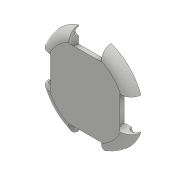
# Autodesk Inventor part: wheel_cover_in
Saved by Autodesk Inventor 2017 (Build 210142000, 142)
## iProperties
Created: 2018-10-27
Part Number: wheel_cover_in
Material: Generic
Document SubType Name: Modeling
Designer: mfans
Density: 1 g/cm^3
Appearance: Default
Author: mfans
Autodesk Inventor part; units mm, degrees
ref_plane "YZ Plane" through (0, 0, 0) normal (1, 0, 0) x (0, 1, 0)
ref_plane "XZ Plane" through (0, 0, 0) normal (0, 1, 0) x (-1, 0, 0)
ref_plane "XY Plane" through (0, 0, 0) normal (0, 0, 1) x (1, 0, 0)
sketch "Sketch1" plane through (0, 0, 0) normal (0, 1, 0) x (-1, 0, 0)
  circle A0 centre (0, 0) radius 30
  dimension "d0" = 60
  constraints: 1 centre point, 1 coincident
  measures "d0" diameter of A0
extrude "Extrusion1" add sketch "Sketch1" against normal blind 6
sketch "Sketch2" plane through (0, 0, 0) normal (0, 1, 0) x (1, 0, 0)
  line L0 (-10, -18) -> (10, -18)
  line L1 (10, -32) -> (-10, -32)
  line L2 (-10, -18) -> (10, -32) construction
  line L3 (10, -18) -> (-10, -32) construction
  arc A0 (-7.5, -25) -> (-12.5, -25) centre (-10, -25) ccw
  arc A1 (12.5, -25) -> (7.5, -25) centre (10, -25) ccw
  line L4 (-12.5, -25) -> (12.5, -25)
  line L5 (-10, -32) -> (-10, -27.5)
  line L6 (-10, -25) -> (-10, -18)
  line L7 (10, -18) -> (10, -25)
  line L8 (10, -27.5) -> (10, -32)
  point P0 (0, 0)
  point P1 (0, -25)
  dimension "d3" = 20
  dimension "d4" = 25
  dimension "d5" = 14
  dimension "d6" = 5
  dimension "d7" = 5
  constraints: 18 end point, 5 parallel, 4 point on circle, 4 point on line, 2 centre point, 2 horizontal, 2 midpoint, 2 perpendicular
  measures "d3" distance of L0.start L0.end
  measures "d4" distance of point (0, 0) point (0, -25)
  measures "d5" distance of L0.end L1.start
  measures "d6" diameter of A0
  measures "d7" diameter of A1
revolve "Revolution1" cut sketch "Sketch2" angle 360 about axis through (-12.5, 0, 25) along (1, 0, 0)
sketch "Sketch3" plane through (0, -6, 0) normal (0, -1, 0) x (1, 0, 0)
  arc A0 (9.04, 28.6056) -> (-9.04, 28.6056) centre (0, 0) ccw projected
  line L0 (-9.04, 28.6056) -> (9.04, 28.6056) projected
  arc A1 (9.04, 28.6056) -> (-9.04, 28.6056) centre (0, 0) ccw projected
extrude "Extrusion2" cut sketch "Sketch3" against normal through all
fillet "Fillet1" radius 6 1 edges at (0, -6, -30)
pattern_circular "Circular Pattern1" count 4 over 360 about axis through (0, -10, 0) along (0, 1, 0) of "Revolution1"
body "Solid1"
